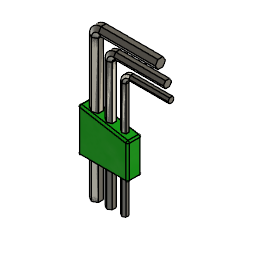
Hex Keys (Autodesk Fusion 360 design; units mm, degrees)
part number: 2026-06-11-09-24-51-850
Autodesk Fusion 360 part; units mm, degrees
sketch "Sketch1" plane through (0, 0, 0) normal (0, 0, 1) x (1, 0, 0)
  line L0 (14.5, -0.866) -> (16, -1.7321)
  line L1 (16, -1.7321) -> (17.5, -0.866)
  line L2 (17.5, -0.866) -> (17.5, 0.866)
  line L3 (17.5, 0.866) -> (16, 1.7321)
  line L4 (16, 1.7321) -> (14.5, 0.866)
  line L5 (14.5, 0.866) -> (14.5, -0.866)
  line L6 (8, 2.3094) -> (6, 1.1547)
  line L7 (6, 1.1547) -> (6, -1.1547)
  line L8 (6, -1.1547) -> (8, -2.3094)
  line L9 (8, -2.3094) -> (10, -1.1547)
  line L10 (10, -1.1547) -> (10, 1.1547)
  line L11 (10, 1.1547) -> (8, 2.3094)
  line L12 (-2.4946, 1.4448) -> (-2.5053, -1.4419)
  line L13 (-2.5053, -1.4419) -> (-0.0107, -2.8946)
  line L14 (-0.0107, -2.8946) -> (2.4946, -1.4605)
  line L15 (2.4946, -1.4605) -> (2.5053, 1.4263)
  line L16 (2.5053, 1.4263) -> (0.0107, 2.8789)
  line L17 (0.0107, 2.8789) -> (-2.4946, 1.4448)
  point P0 (16, 0)
  point P1 (8, 0)
  point P2 (0, -0.0078)
  dimension "d1" = 3
  dimension "d2" = 4
  dimension "d3" = 5
  dimension "d4" = 8
  dimension "d5" = 8
  constraint vertical origin P2
  constraint horizontal origin P0
  constraint horizontal origin P1
  measures "d1" distance of L2 L5
  measures "d2" distance of L7 L10
  measures "d3" distance of L12 L15
  measures "d4" distance of origin P1
  measures "d5" distance of P0 P1
sketch "Sketch3" plane through (0, 0, 0) normal (0, 1, 0) x (1, 0, 0)
  line L0 (0, -80) -> (0, 0)
  line L1 (8, 0) -> (8, -72)
  line L2 (16, 0) -> (16, -65)
  line L3 (4, -84) -> (36, -84)
  line L4 (12, -76) -> (40, -76)
  line L5 (20, -69) -> (42, -69)
  arc A0 (0, -80) -> (4, -84) centre (4, -80) ccw
  arc A1 (8, -72) -> (12, -76) centre (12, -72) ccw
  arc A2 (16, -65) -> (20, -69) centre (20, -65) ccw
  point P0 (2.4946, 0)
  point P1 (10, 0)
  point P2 (17.5, 0)
  point P3 (8, 0)
  point P4 (16, 0)
  dimension "d6" = 8
  dimension "d7" = 8
  dimension "d9" = 8
  dimension "d10" = 80
  dimension "d11" = 72
  dimension "d12" = 65
  dimension "d13" = 32
  dimension "d14" = 28
  dimension "d15" = 22
  constraint coincident L0.end origin
  constraint coincident P3 L1.start
  constraint tangent L1 A1
  constraint coincident P4 L2.start
  constraint tangent L2 A2
  constraint vertical L2
  constraint vertical L1
  constraint vertical L0
  constraint horizontal L3
  constraint horizontal L4
  constraint parallel L4 L5
  constraint tangent L3 A0
  constraint tangent L4 A1
  constraint tangent L5 A2
  constraint tangent L0 A0
  measures "d6" diameter of A1
  measures "d7" diameter of A0
  measures "d9" diameter of A2
  measures "d10" vertical distance of A0.centre P0
  measures "d11" vertical distance of A1.centre P1
  measures "d12" vertical distance of A2.centre P2
  measures "d13" distance of L3.start L3.end
  measures "d14" distance of L4.start L4.end
  measures "d15" distance of L5.start L5.end
sweep "Sweep1" add profiles "Sketch1" path "Sketch3" along L3 A0 L0 section 1 contours L12 L13 L14 L15 L16 L17 makes body 1
sweep "Sweep2" add profiles "Sketch1" path "Sketch3" along L1 A1 L4 section 1 contours L6 L7 L8 L9 L10 L11 separate body makes body 2
sweep "Sweep3" add profiles "Sketch1" path "Sketch3" along L2 A2 L5 section 1 contours L0 L1 L2 L3 L4 L5 separate body makes body 3
sketch "Sketch4" plane through (0, 0, 0) normal (0, 1, 0) x (1, 0, 0)
  line L0 (-6.5053, -45) -> (-6.5053, -20)
  line L1 (17.5, 0) -> (17.5, -65)
  line L2 (-6.5053, -20) -> (21.5, -20)
  line L3 (21.5, -20) -> (21.5, -40)
  line L4 (21.5, -40) -> (-6.5053, -45)
  line L5 (-2.5053, 0) -> (-2.5053, -80)
  dimension "d34" = 20
  dimension "d35" = 25
  dimension "d36" = 20
  dimension "d37" = 4
  dimension "d38" = 4
  constraint vertical L0
  constraint perpendicular L1 L2
  constraint perpendicular L2 L3
  measures "d34" vertical distance of origin L0.end
  measures "d35" distance of L0.start L0.end
  measures "d36" distance of L2.end L3.end
  measures "d37" distance of L0.start L5
  measures "d38" distance of L1 L3.end
extrude "Extrude1" add sketch "Sketch4" along normal mid plane 8 separate body makes body 4
fillet "Fillet1" radius 1 12 edges at (7.4973, -4, 42.5) (7.4973, 4, 42.5) (-6.5053, 0, 45) (21.5, 0, 40) (21.5, -4, 30) (21.5, 4, 30) (7.4973, -4, 20) (-6.5053, -4, 32.5) (21.5, 0, 20) (7.4973, 4, 20) (-6.5053, 0, 20) (-6.5053, 4, 32.5) on bodies 4
combine "Combine1" operation add target body 4 tool bodies 1 2 3 keep tools
